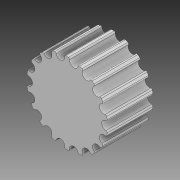
# Autodesk Inventor part: Timing Pulley Generator
Saved by Autodesk Inventor 2022 (Build 260153000, 153)
## iProperties
Created: 2022-01-03
Part Number: Timing Pulley Generator
Material: Generic
Document SubType Name: Modeling
Density: 1 g/cm^3
Appearance: Default
Autodesk Inventor part; units mm, degrees
ref_plane "YZ Plane" through (0, 0, 0) normal (1, 0, 0) x (0, 1, 0)
ref_plane "XZ Plane" through (0, 0, 0) normal (0, 1, 0) x (-1, 0, 0)
ref_plane "XY Plane" through (0, 0, 0) normal (0, 0, 1) x (1, 0, 0)
sketch "Sketch1" plane through (0, 0, 0) normal (0, 0, 1) x (1, 0, 0)
  circle A0 centre (0, 0) radius 8.5944
  dimension "d0" = 17.1887
  constraints: 1 centre point, 1 coincident
  measures "d0" diameter of A0
extrude "Base" add sketch "Sketch1" along normal mid plane 9
sketch "Sketch2" plane through (0, 0, 4.5) normal (0, 0, 1) x (1, 0, 0)
  arc A0 (-0.7044, 7.6922) -> (0, 7.7244) centre (0, 0) ccw
  arc A1 (-0.238, 7.2151) -> (-0.7044, 7.6922) centre (-0.6652, 7.264) ccw
  arc A2 (-0.238, 7.2151) -> (0.9836, 5.5783) centre (1.2423, 7.0457) ccw
  circle A3 centre (0, 0) radius 8.5944 construction
  line L0 (0, 0) -> (0, 7.7244) construction
  line L1 (1.2423, 7.0457) -> (0, 0) construction
  line L2 (-2.3111, 9.1345) -> (5.2959, 7.7931) construction
  line L3 (1.4924, 8.4638) -> (0.9836, 5.5783)
  arc A4 (1.4924, 8.4638) -> (0, 8.5944) centre (0, 0) ccw
  line L4 (0, 7.7244) -> (0, 8.5944)
  dimension "d3" = 0.43
  dimension "d4" = 1.49
  dimension "d5" = 0.87
  dimension "d6" = 2.93
  dimension "d7" = 10
  constraints: 10 end point, 10 point on circle, 4 centre point, 3 tangent, 2 coincident, 2 vertical, 2 vertical alignment, 1 equal length, 1 midpoint, 1 perpendicular, 1 point on line
  measures "d3" radius of A1
  measures "d4" radius of A2
  measures "d5" distance of L0.end L4.end
  measures "d6" distance of L3.start L3.end
  measures "d7" angle of L1 L0
extrude "HTD Tooth" [suppressed]
mirror "HTD Tooth Mirror" [suppressed]
pattern_circular "HTD Pattern" [suppressed]
sketch "Sketch3" plane through (0, 0, 4.5) normal (0, 0, 1) x (1, 0, 0)
  arc A0 (0.2512, 7.9604) -> (0, 7.9644) centre (0, 0) ccw
  arc A1 (0.4909, 7.6758) -> (0.2512, 7.9604) centre (0.2433, 7.7105) ccw
  arc A2 (0.4909, 7.6758) -> (1.185, 6.7207) centre (1.3326, 7.5578) ccw
  line L0 (0, 0) -> (0, 7.9644) construction
  line L1 (1.3326, 7.5578) -> (0, 0) construction
  line L2 (-2.4293, 9.1553) -> (5.4141, 7.7723) construction
  line L3 (1.4924, 8.4638) -> (1.185, 6.7207)
  arc A3 (1.4924, 8.4638) -> (0, 8.5944) centre (0, 0) ccw
  line L4 (0, 7.9644) -> (0, 8.5944)
  circle A4 centre (0, 0) radius 8.5944 construction
  dimension "d13" = 0.25
  dimension "d14" = 0.85
  dimension "d15" = 0.63
  dimension "d16" = 1.77
  dimension "d17" = 10
  constraints: 10 end point, 8 point on circle, 4 centre point, 2 coincident, 2 tangent, 2 vertical, 2 vertical alignment, 1 collinear, 1 concentric, 1 equal length, 1 midpoint, 1 perpendicular, 1 point on line
  measures "d13" radius of A1
  measures "d14" radius of A2
  measures "d15" distance of L0.end L4.end
  measures "d16" distance of L3.start L3.end
  measures "d17" angle of L1 L0
extrude "GT2 Tooth" cut sketch "Sketch3" against normal through all
mirror "GT2 Tooth Mirror" about plane through (0, 0, 0) normal (1, 0, 0) of "GT2 Tooth"
pattern_circular "Circular Pattern2" count 18 over 360 about axis through (0, 0, -10) along (0, 0, 1) of "GT2 Tooth", "GT2 Tooth Mirror"
equation "\"d0\" = Pitch_Diameter"
equation "\"d1\" = Width"
equation "\"d3\" = HTD_Root_Fillet_Rad"
equation "\"d4\" = HTD_Tooth_Rad"
equation "\"d5\" = HTD_Root_to_Pitch_Diameter"
equation "\"d6\" = HTD_Root_to_Pitch_Diameter + HTD_Belt_Tooth_Height"
equation "\"d8\" = Width"
equation "\"d13\" = GT2_Root_Fillet_Rad"
equation "\"d14\" = GT2_Tooth_Rad"
equation "\"d15\" = GT2_Root_to_Pitch_Diameter"
equation "\"d16\" = GT2_Root_to_Pitch_Diameter + GT2_Belt_Tooth_Height"
equation "\"Pitch\" = 3"
equation "\"Width\" = 9"
equation "\"HTD_Root_Fillet_Rad\" = 0.43"
equation "\"HTD_Tooth_Rad\" = 1.49"
equation "\"HTD_Belt_Height\" = 3.8"
equation "\"HTD_Belt_Tooth_Height\" = 2.06"
equation "\"HTD_Root_to_Pitch_Diameter\" = -0.5 * HTD_Belt_Tooth_Height + 0.5 * HTD_Belt_Height"
equation "\"GT2_Root_Fillet_Rad\" = 0.25"
equation "\"GT2_Tooth_Rad\" = 0.85"
equation "\"GT2_Root_to_Pitch_Diameter\" = -0.5 * GT2_Belt_Tooth_Height + 0.5 * GT2_Belt_Height"
equation "\"GT2_Belt_Tooth_Height\" = 1.14"
equation "\"GT2_Belt_Height\" = 2.4"
equation "\"Pitch_Diameter\" = 17.188734"
body "Solid1"
